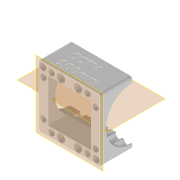
# Autodesk Inventor part: 11_Cube_Berrybase_CCTV_100mm_Lens_Cube_half
Saved by Autodesk Inventor 2022 (Build 260153000, 153)
## iProperties
Created: 2023-01-17
Part Number: 11_Cube_Berrybase_CCTV_100mm_Lens_Cube_half
Material: Generisch
Document SubType Name: Modeling
Designer: diederichbenedict
Density: 1 g/cm^3
Appearance: Vorgabe
Author: diederichbenedict
Autodesk Inventor part; units mm, degrees
ref_plane "YZ Plane" through (0, 0, 0) normal (1, 0, 0) x (0, 1, 0)
ref_plane "XZ Plane" through (0, 0, 0) normal (0, 1, 0) x (-1, 0, 0)
ref_plane "Arbeitsebene1" through (0, 0, 0) normal (0, 0, 1) x (1, 0, 0)
ref_plane "Arbeitsebene2" through (24.9, -0.1027, -25.0973) normal (0, 1, 0) x (-1, 0, 0)
sketch "Skizze3" plane through (0, 0, 0) normal (0, 0, 1) x (1, 0, 0)
  circle A0 centre (20.71, -14.2755) radius 2.475 projected
  circle A1 centre (14.3, 20.7345) radius 2.475 projected
  circle A2 centre (-20.71, 14.3245) radius 2.475 projected
  circle A3 centre (-14.3, -20.6855) radius 2.475 projected
  circle A4 centre (14.3, -20.6855) radius 2.475 projected
  circle A5 centre (-20.71, -14.2755) radius 2.475 projected
  circle A6 centre (-14.3, 20.7345) radius 2.475 projected
  circle A7 centre (20.71, 14.3245) radius 2.475 projected
  line L0 (-17.02, 17.0445) -> (-17.02, -16.9955) projected
  line L1 (-17.02, -16.9955) -> (17.02, -16.9955) projected
  line L2 (17.02, -16.9955) -> (17.02, 17.0445) projected
  line L3 (17.02, 17.0445) -> (-17.02, 17.0445) projected
  circle A8 centre (-21.25, 21.2745) radius 2.75 projected
  circle A9 centre (21.25, -21.2255) radius 2.75 projected
  arc A10 (-22.9, 24.4245) -> (-24.4, 22.9245) centre (-22.9, 22.9245) ccw projected
  line L4 (22.9, 24.4245) -> (-22.9, 24.4245) projected
  arc A11 (24.4, 22.9245) -> (22.9, 24.4245) centre (22.9, 22.9245) ccw projected
  line L5 (24.4, -22.8755) -> (24.4, 22.9245) projected
  arc A12 (22.9, -24.3755) -> (24.4, -22.8755) centre (22.9, -22.8755) ccw projected
  line L6 (-22.9, -24.3755) -> (22.9, -24.3755) projected
  arc A13 (-24.4, -22.8755) -> (-22.9, -24.3755) centre (-22.9, -22.8755) ccw projected
  line L7 (-24.4, 22.9245) -> (-24.4, -22.8755) projected
  arc A14 (24.9, 22.9) -> (22.9, 24.9) centre (22.9, 22.9) ccw projected
  arc A15 (-22.9, 24.9) -> (-24.8755, 22.9245) centre (-22.9, 22.9245) ccw
  line L8 (-24.8755, 22.9245) -> (-24.8755, -22.8755)
  arc A16 (-24.8755, -22.8755) -> (-22.9, -24.8509) centre (-22.9, -22.8755) ccw
  line L9 (-22.9, -24.8509) -> (22.9, -24.8509)
  arc A17 (22.9, -24.8509) -> (24.8755, -22.8755) centre (22.9, -22.8755) ccw
  line L10 (24.8755, -22.8755) -> (24.8755, 22.9245)
  arc A18 (24.8755, 22.9245) -> (22.9, 24.9) centre (22.9, 22.9245) ccw
  line L11 (22.9, 24.9) -> (-22.9, 24.9)
  point P0 (0, 0)
  constraints: 8 end point, 8 point on circle, 4 centre point, 7 other
ref_plane "Arbeitsebene3" through (-43.875, -23.2027, -25.0973) normal (0, 0, 1) x (1, 0, 0)
extrude "Extrusion1" add sketch "Skizze3" against normal up to surface (25.0973 mm away) contours L4 A11 L5 A12 L6 A13 L7 A10 | L11 A18 L10 A17 L9 A16 L8 A15
sketch "Skizze2" plane through (24.9, -0.1027, -25.0973) normal (0, 1, 0) x (-1, 0, 0)
  line L0 (65.5, -19.5) -> (13.5, -19.5)
  line L1 (13.5, -19.5) -> (9.5, -21)
  line L2 (9.5, -21) -> (0, -21)
  line L3 (0, -21) -> (0, 0)
  line L4 (0, 0) -> (65.5, 0)
  line L5 (65.5, 0) -> (65.5, -19.5)
  line L6 (-13.1, 0) -> (78.6, 0)
  point P0 (24.9, 25.0973)
  point P1 (7.88, -21.1827)
  constraints: 14 end point, 3 horizontal, 2 perpendicular, 1 point on line, 1 vertical, 8 other
revolve "Umdrehung1" cut sketch "Skizze2" angle 360 about axis through (24.9, -0.1027, -25.0973) along (-1, 0, 0)
sketch "Skizze4" plane through (0, 0, 0) normal (0, 0, 1) x (1, 0, 0)
  circle A0 centre (20.71, 14.3) radius 2.475 projected
  circle A1 centre (14.3, -20.71) radius 2.475 projected
  circle A2 centre (-20.71, -14.3) radius 2.475 projected
  circle A3 centre (-14.3, 20.71) radius 2.475 projected
  circle A4 centre (14.3, 20.71) radius 2.475 projected
  circle A5 centre (-20.71, 14.3) radius 2.475 projected
  circle A6 centre (-14.3, -20.71) radius 2.475 projected
  circle A7 centre (20.71, -14.3) radius 2.475 projected
  line L0 (-17.02, -17.02) -> (-17.02, 17.02) projected
  line L1 (-17.02, 17.02) -> (17.02, 17.02) projected
  line L2 (17.02, 17.02) -> (17.02, -17.02) projected
  line L3 (17.02, -17.02) -> (-17.02, -17.02) projected
  circle A8 centre (-21.25, -21.25) radius 2.75 projected
  circle A9 centre (21.25, 21.25) radius 2.75 projected
  arc A10 (-24.4, -22.9) -> (-22.9, -24.4) centre (-22.9, -22.9) ccw projected
  line L4 (22.9, -24.4) -> (-22.9, -24.4) projected
  arc A11 (22.9, -24.4) -> (24.4, -22.9) centre (22.9, -22.9) ccw projected
  line L5 (24.4, 22.9) -> (24.4, -22.9) projected
  arc A12 (24.4, 22.9) -> (22.9, 24.4) centre (22.9, 22.9) ccw projected
  line L6 (-22.9, 24.4) -> (22.9, 24.4) projected
  arc A13 (-22.9, 24.4) -> (-24.4, 22.9) centre (-22.9, 22.9) ccw projected
  line L7 (-24.4, -22.9) -> (-24.4, 22.9) projected
  circle A14 centre (6.8, -20.71) radius 1.4
  circle A15 centre (-6.8, -20.71) radius 1.4
  point P0 (0, 0)
  dimension "d3" = 2.8
  dimension "d4" = 2.8
  dimension "d5" = 7.5
  dimension "d6" = 7.5
  constraints: 2 centre point
  measures "d3" diameter of A14
  measures "d4" diameter of A15
  measures "d5" distance of A14.centre A1.centre
  measures "d6" distance of A6.centre A15.centre
hole "Bohrung1" at (6.8, -20.71, 0) at (-6.8, -20.71, 0) direction (0, 0, -1) diameter 2.8 end through all counterbore diameter 6.5 counterbore depth 10
mirror "Spiegeln1" about plane through (24.9, -0.1027, -25.0973) normal (0, 1, 0) of "Bohrung1"
fillet "Rundung1" radius 1 8 edges at (24.2969, 24.3214, 0) (0, 24.9, 0) (-24.2969, 24.3214, 0) (-24.8755, 0.0245, 0) (-24.2969, -24.2723, 0) (0, -24.8509, 0) (24.2969, -24.2723, 0) (24.8755, 0.0245, 0)
sketch "Skizze5" plane through (-22.9, 24.9, -25.0973) normal (0, 1, 0) x (1, 0, 0)
  line L0 (7.1527, -5.0272) -> (36.083, -5.0272) construction
  line L1 (36.083, -5.0272) -> (36.083, -3.8859) construction
  line L2 (36.083, -3.8859) -> (7.1527, -3.8859) construction
  line L3 (7.1527, -3.8859) -> (7.1527, -5.0272) construction
  spline S0 degree 2 poles (10.4153, -11.3645) (9.0411, -11.3645) (7.4296, -9.7035) (7.4296, -8.2008) knots 0 0 0 1 2 2 2
  spline S1 degree 2 poles (7.4296, -8.2008) (7.4296, -6.7524) (9.046, -5.0272) (10.4202, -5.0272) knots 0 0 0 1 2 2 2
  spline S2 degree 2 poles (10.4202, -5.0272) (10.7811, -5.0272) (11.3644, -5.1112) (11.6313, -5.1805) knots 0 0 0 1 2 2 2
  spline S3 degree 2 poles (11.6313, -5.1805) (11.839, -5.2447) (12.3283, -5.4573) (12.4816, -5.5364) knots 0 0 0 1 2 2 2
  line L4 (12.4816, -5.5364) -> (12.4816, -6.9897)
  line L5 (12.4816, -6.9897) -> (12.3283, -6.9897)
  spline S4 degree 2 poles (12.3283, -6.9897) (12.2146, -6.8908) (11.8785, -6.614) (11.6659, -6.4855) knots 0 0 0 1 2 2 2
  spline S5 degree 2 poles (11.6659, -6.4855) (11.4534, -6.352) (10.9442, -6.1691) (10.6625, -6.1691) knots 0 0 0 1 2 2 2
  spline S6 degree 2 poles (10.6625, -6.1691) (10.3313, -6.1691) (9.7825, -6.3767) (9.5304, -6.6387) knots 0 0 0 1 2 2 2
  spline S7 degree 2 poles (9.5304, -6.6387) (9.3031, -6.8711) (9.0114, -7.6669) (9.0114, -8.2057) knots 0 0 0 1 2 2 2
  spline S8 degree 2 poles (9.0114, -8.2057) (9.0114, -8.7742) (9.3129, -9.5503) (9.5601, -9.7876) knots 0 0 0 1 2 2 2
  spline S9 degree 2 poles (9.5601, -9.7876) (9.7974, -10.0199) (10.3807, -10.2226) (10.6723, -10.2226) knots 0 0 0 1 2 2 2
  spline S10 degree 2 poles (10.6723, -10.2226) (10.9739, -10.2226) (11.5226, -10.0199) (11.7104, -9.8963) knots 0 0 0 1 2 2 2
  spline S11 degree 2 poles (11.7104, -9.8963) (11.918, -9.7728) (12.2295, -9.5108) (12.3432, -9.407) knots 0 0 0 1 2 2 2
  line L6 (12.3432, -9.407) -> (12.4816, -9.407)
  line L7 (12.4816, -9.407) -> (12.4816, -10.8405)
  spline S12 degree 2 poles (12.4816, -10.8405) (12.3135, -10.9196) (11.8736, -11.1173) (11.6363, -11.1865) knots 0 0 0 1 2 2 2
  spline S13 degree 2 poles (11.6363, -11.1865) (11.3496, -11.2755) (10.8503, -11.3645) (10.4153, -11.3645) knots 0 0 0 1 2 2 2
  spline S14 degree 2 poles (16.016, -11.3645) (14.6418, -11.3645) (13.0303, -9.7035) (13.0303, -8.2008) knots 0 0 0 1 2 2 2
  spline S15 degree 2 poles (13.0303, -8.2008) (13.0303, -6.7524) (14.6467, -5.0272) (16.021, -5.0272) knots 0 0 0 1 2 2 2
  spline S16 degree 2 poles (16.021, -5.0272) (16.3818, -5.0272) (16.9651, -5.1112) (17.2321, -5.1805) knots 0 0 0 1 2 2 2
  spline S17 degree 2 poles (17.2321, -5.1805) (17.4397, -5.2447) (17.9291, -5.4573) (18.0823, -5.5364) knots 0 0 0 1 2 2 2
  line L8 (18.0823, -5.5364) -> (18.0823, -6.9897)
  line L9 (18.0823, -6.9897) -> (17.9291, -6.9897)
  spline S18 degree 2 poles (17.9291, -6.9897) (17.8154, -6.8908) (17.4792, -6.614) (17.2667, -6.4855) knots 0 0 0 1 2 2 2
  spline S19 degree 2 poles (17.2667, -6.4855) (17.0541, -6.352) (16.5449, -6.1691) (16.2632, -6.1691) knots 0 0 0 1 2 2 2
  spline S20 degree 2 poles (16.2632, -6.1691) (15.932, -6.1691) (15.3833, -6.3767) (15.1312, -6.6387) knots 0 0 0 1 2 2 2
  spline S21 degree 2 poles (15.1312, -6.6387) (14.9038, -6.8711) (14.6121, -7.6669) (14.6121, -8.2057) knots 0 0 0 1 2 2 2
  spline S22 degree 2 poles (14.6121, -8.2057) (14.6121, -8.7742) (14.9137, -9.5503) (15.1608, -9.7876) knots 0 0 0 1 2 2 2
  spline S23 degree 2 poles (15.1608, -9.7876) (15.3981, -10.0199) (15.9814, -10.2226) (16.2731, -10.2226) knots 0 0 0 1 2 2 2
  spline S24 degree 2 poles (16.2731, -10.2226) (16.5746, -10.2226) (17.1233, -10.0199) (17.3112, -9.8963) knots 0 0 0 1 2 2 2
  spline S25 degree 2 poles (17.3112, -9.8963) (17.5188, -9.7728) (17.8302, -9.5108) (17.9439, -9.407) knots 0 0 0 1 2 2 2
  line L10 (17.9439, -9.407) -> (18.0823, -9.407)
  line L11 (18.0823, -9.407) -> (18.0823, -10.8405)
  spline S26 degree 2 poles (18.0823, -10.8405) (17.9142, -10.9196) (17.4743, -11.1173) (17.237, -11.1865) knots 0 0 0 1 2 2 2
  spline S27 degree 2 poles (17.237, -11.1865) (16.9503, -11.2755) (16.451, -11.3645) (16.016, -11.3645) knots 0 0 0 1 2 2 2
  line L12 (20.1585, -11.2458) -> (20.1585, -6.3075)
  line L13 (20.1585, -6.3075) -> (18.3542, -6.3075)
  line L14 (18.3542, -6.3075) -> (18.3542, -5.1458)
  line L15 (18.3542, -5.1458) -> (23.4952, -5.1458)
  line L16 (23.4952, -5.1458) -> (23.4952, -6.3075)
  line L17 (23.4952, -6.3075) -> (21.6909, -6.3075)
  line L18 (21.6909, -6.3075) -> (21.6909, -11.2458)
  line L19 (21.6909, -11.2458) -> (20.1585, -11.2458)
  line L20 (29.2146, -5.1458) -> (27.1186, -11.2458)
  line L21 (27.1186, -11.2458) -> (25.5219, -11.2458)
  line L22 (25.5219, -11.2458) -> (23.426, -5.1458)
  line L23 (23.426, -5.1458) -> (25.0128, -5.1458)
  line L24 (25.0128, -5.1458) -> (26.3425, -9.2834)
  line L25 (26.3425, -9.2834) -> (27.6673, -5.1458)
  line L26 (27.6673, -5.1458) -> (29.2146, -5.1458)
  line L27 (11.9823, -21.2893) -> (7.9535, -21.2893)
  line L28 (7.9535, -21.2893) -> (7.9535, -20.2265)
  line L29 (7.9535, -20.2265) -> (9.2388, -20.2265)
  line L30 (9.2388, -20.2265) -> (9.2388, -16.9986)
  line L31 (9.2388, -16.9986) -> (7.9535, -16.9986)
  line L32 (7.9535, -16.9986) -> (7.9535, -16.005)
  spline S28 degree 2 poles (7.9535, -16.005) (8.2353, -16.005) (8.7939, -15.9308) (8.962, -15.8517) knots 0 0 0 1 2 2 2
  spline S29 degree 2 poles (8.962, -15.8517) (9.1548, -15.7529) (9.3723, -15.4217) (9.392, -15.1745) knots 0 0 0 1 2 2 2
  line L33 (9.392, -15.1745) -> (10.7267, -15.1745)
  line L34 (10.7267, -15.1745) -> (10.7267, -20.2265)
  line L35 (10.7267, -20.2265) -> (11.9823, -20.2265)
  line L36 (11.9823, -20.2265) -> (11.9823, -21.2893)
  spline S30 degree 2 poles (17.5188, -18.2393) (17.5188, -19.0303) (17.2667, -20.2166) (16.9849, -20.6171) knots 0 0 0 1 2 2 2
  spline S31 degree 2 poles (16.9849, -20.6171) (16.7081, -21.0125) (15.8133, -21.4179) (15.1707, -21.4179) knots 0 0 0 1 2 2 2
  spline S32 degree 2 poles (15.1707, -21.4179) (14.5231, -21.4179) (13.6334, -21.0125) (13.3516, -20.6072) knots 0 0 0 1 2 2 2
  spline S33 degree 2 poles (13.3516, -20.6072) (13.0698, -20.2068) (12.8177, -19.0303) (12.8177, -18.2393) knots 0 0 0 1 2 2 2
  spline S34 degree 2 poles (12.8177, -18.2393) (12.8177, -17.4286) (13.0698, -16.2818) (13.3565, -15.8666) knots 0 0 0 1 2 2 2
  spline S35 degree 2 poles (13.3565, -15.8666) (13.6432, -15.4612) (14.5479, -15.0658) (15.1707, -15.0658) knots 0 0 0 1 2 2 2
  spline S36 degree 2 poles (15.1707, -15.0658) (15.8282, -15.0658) (16.7081, -15.481) (16.9898, -15.8913) knots 0 0 0 1 2 2 2
  spline S37 degree 2 poles (16.9898, -15.8913) (17.2667, -16.2917) (17.5188, -17.4731) (17.5188, -18.2393) knots 0 0 0 1 2 2 2
  spline S38 degree 2 poles (15.9814, -18.2393) (15.9814, -17.1073) (15.6107, -16.1928) (15.1707, -16.1928) knots 0 0 0 1 2 2 2
  spline S39 degree 2 poles (15.1707, -16.1928) (14.7308, -16.1928) (14.3551, -17.1073) (14.3551, -18.2443) knots 0 0 0 1 2 2 2
  spline S40 degree 2 poles (14.3551, -18.2443) (14.3551, -19.3615) (14.7308, -20.2908) (15.1707, -20.2908) knots 0 0 0 1 2 2 2
  spline S41 degree 2 poles (15.1707, -20.2908) (15.6057, -20.2908) (15.9814, -19.3615) (15.9814, -18.2393) knots 0 0 0 1 2 2 2
  spline S42 degree 2 poles (22.8625, -18.2393) (22.8625, -19.0303) (22.6103, -20.2166) (22.3286, -20.6171) knots 0 0 0 1 2 2 2
  spline S43 degree 2 poles (22.3286, -20.6171) (22.0518, -21.0125) (21.157, -21.4179) (20.5144, -21.4179) knots 0 0 0 1 2 2 2
  spline S44 degree 2 poles (20.5144, -21.4179) (19.8668, -21.4179) (18.977, -21.0125) (18.6953, -20.6072) knots 0 0 0 1 2 2 2
  spline S45 degree 2 poles (18.6953, -20.6072) (18.4135, -20.2068) (18.1614, -19.0303) (18.1614, -18.2393) knots 0 0 0 1 2 2 2
  spline S46 degree 2 poles (18.1614, -18.2393) (18.1614, -17.4286) (18.4135, -16.2818) (18.7002, -15.8666) knots 0 0 0 1 2 2 2
  spline S47 degree 2 poles (18.7002, -15.8666) (18.9869, -15.4612) (19.8915, -15.0658) (20.5144, -15.0658) knots 0 0 0 1 2 2 2
  spline S48 degree 2 poles (20.5144, -15.0658) (21.1719, -15.0658) (22.0518, -15.481) (22.3335, -15.8913) knots 0 0 0 1 2 2 2
  spline S49 degree 2 poles (22.3335, -15.8913) (22.6103, -16.2917) (22.8625, -17.4731) (22.8625, -18.2393) knots 0 0 0 1 2 2 2
  spline S50 degree 2 poles (21.3251, -18.2393) (21.3251, -17.1073) (20.9543, -16.1928) (20.5144, -16.1928) knots 0 0 0 1 2 2 2
  spline S51 degree 2 poles (20.5144, -16.1928) (20.0744, -16.1928) (19.6988, -17.1073) (19.6988, -18.2443) knots 0 0 0 1 2 2 2
  spline S52 degree 2 poles (19.6988, -18.2443) (19.6988, -19.3615) (20.0744, -20.2908) (20.5144, -20.2908) knots 0 0 0 1 2 2 2
  spline S53 degree 2 poles (20.5144, -20.2908) (20.9494, -20.2908) (21.3251, -19.3615) (21.3251, -18.2393) knots 0 0 0 1 2 2 2
  line L37 (29.2244, -21.2893) -> (29.2244, -18.9907)
  spline S54 degree 2 poles (29.2244, -18.9907) (29.2244, -18.6496) (29.1997, -18.185) (29.1404, -18.0367) knots 0 0 0 1 2 2 2
  spline S55 degree 2 poles (29.1404, -18.0367) (29.0761, -17.8884) (28.8191, -17.7549) (28.5868, -17.7549) knots 0 0 0 1 2 2 2
  spline S56 degree 2 poles (28.5868, -17.7549) (28.4236, -17.7549) (28.1073, -17.8983) (27.9194, -18.0317) knots 0 0 0 1 2 2 2
  line L38 (27.9194, -18.0317) -> (27.9194, -21.2893)
  line L39 (27.9194, -21.2893) -> (26.476, -21.2893)
  line L40 (26.476, -21.2893) -> (26.476, -18.9907)
  spline S57 degree 2 poles (26.476, -18.9907) (26.476, -18.6546) (26.4463, -18.185) (26.387, -18.0367) knots 0 0 0 1 2 2 2
  spline S58 degree 2 poles (26.387, -18.0367) (26.3227, -17.8884) (26.0657, -17.7549) (25.8334, -17.7549) knots 0 0 0 1 2 2 2
  spline S59 degree 2 poles (25.8334, -17.7549) (25.6603, -17.7549) (25.3193, -17.918) (25.1611, -18.0317) knots 0 0 0 1 2 2 2
  line L41 (25.1611, -18.0317) -> (25.1611, -21.2893)
  line L42 (25.1611, -21.2893) -> (23.7275, -21.2893)
  line L43 (23.7275, -21.2893) -> (23.7275, -16.6872)
  line L44 (23.7275, -16.6872) -> (25.1611, -16.6872)
  line L45 (25.1611, -16.6872) -> (25.1611, -17.1963)
  spline S60 degree 2 poles (25.1611, -17.1963) (25.512, -16.8997) (26.1398, -16.5636) (26.5304, -16.5636) knots 0 0 0 1 2 2 2
  spline S61 degree 2 poles (26.5304, -16.5636) (26.9505, -16.5636) (27.5932, -16.964) (27.7612, -17.3644) knots 0 0 0 1 2 2 2
  spline S62 degree 2 poles (27.7612, -17.3644) (28.1715, -16.9788) (28.9031, -16.5636) (29.2788, -16.5636) knots 0 0 0 1 2 2 2
  spline S63 degree 2 poles (29.2788, -16.5636) (29.6001, -16.5636) (30.1093, -16.7662) (30.2823, -16.9739) knots 0 0 0 1 2 2 2
  spline S64 degree 2 poles (30.2823, -16.9739) (30.4751, -17.1963) (30.6679, -17.8043) (30.6679, -18.2937) knots 0 0 0 1 2 2 2
  line L46 (30.6679, -18.2937) -> (30.6679, -21.2893)
  line L47 (30.6679, -21.2893) -> (29.2244, -21.2893)
  line L48 (37.2227, -21.2893) -> (37.2227, -18.9907)
  spline S65 degree 2 poles (37.2227, -18.9907) (37.2227, -18.6496) (37.1979, -18.185) (37.1386, -18.0367) knots 0 0 0 1 2 2 2
  spline S66 degree 2 poles (37.1386, -18.0367) (37.0744, -17.8884) (36.8173, -17.7549) (36.585, -17.7549) knots 0 0 0 1 2 2 2
  spline S67 degree 2 poles (36.585, -17.7549) (36.4219, -17.7549) (36.1055, -17.8983) (35.9176, -18.0317) knots 0 0 0 1 2 2 2
  line L49 (35.9176, -18.0317) -> (35.9176, -21.2893)
  line L50 (35.9176, -21.2893) -> (34.4742, -21.2893)
  line L51 (34.4742, -21.2893) -> (34.4742, -18.9907)
  spline S68 degree 2 poles (34.4742, -18.9907) (34.4742, -18.6546) (34.4445, -18.185) (34.3852, -18.0367) knots 0 0 0 1 2 2 2
  spline S69 degree 2 poles (34.3852, -18.0367) (34.321, -17.8884) (34.0639, -17.7549) (33.8316, -17.7549) knots 0 0 0 1 2 2 2
  spline S70 degree 2 poles (33.8316, -17.7549) (33.6586, -17.7549) (33.3175, -17.918) (33.1593, -18.0317) knots 0 0 0 1 2 2 2
  line L52 (33.1593, -18.0317) -> (33.1593, -21.2893)
  line L53 (33.1593, -21.2893) -> (31.7257, -21.2893)
  line L54 (31.7257, -21.2893) -> (31.7257, -16.6872)
  line L55 (31.7257, -16.6872) -> (33.1593, -16.6872)
  line L56 (33.1593, -16.6872) -> (33.1593, -17.1963)
  spline S71 degree 2 poles (33.1593, -17.1963) (33.5103, -16.8997) (34.1381, -16.5636) (34.5286, -16.5636) knots 0 0 0 1 2 2 2
  spline S72 degree 2 poles (34.5286, -16.5636) (34.9488, -16.5636) (35.5914, -16.964) (35.7595, -17.3644) knots 0 0 0 1 2 2 2
  spline S73 degree 2 poles (35.7595, -17.3644) (36.1697, -16.9788) (36.9014, -16.5636) (37.277, -16.5636) knots 0 0 0 1 2 2 2
  spline S74 degree 2 poles (37.277, -16.5636) (37.5984, -16.5636) (38.1075, -16.7662) (38.2805, -16.9739) knots 0 0 0 1 2 2 2
  spline S75 degree 2 poles (38.2805, -16.9739) (38.4733, -17.1963) (38.6661, -17.8043) (38.6661, -18.2937) knots 0 0 0 1 2 2 2
  line L57 (38.6661, -18.2937) -> (38.6661, -21.2893)
  line L58 (38.6661, -21.2893) -> (37.2227, -21.2893)
  point P0 (22.9, -25.0973)
  constraints: 2 other
extrude "Extrusion2" cut sketch "Skizze5" against normal blind 0.5
